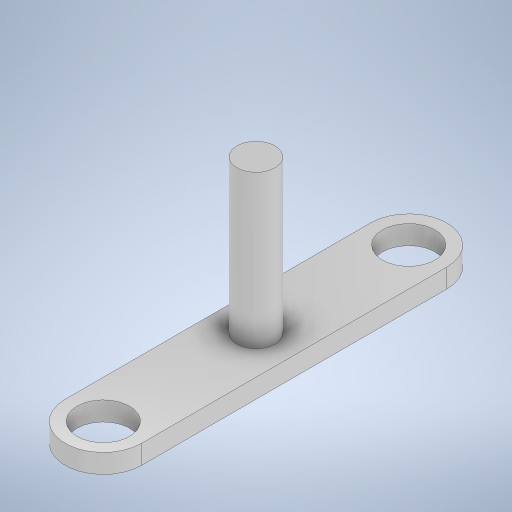
# Autodesk Inventor part: Torqueing_Bar
Saved by Autodesk Inventor 2024 (Build 280153000, 153)
## iProperties
Created: 2023-10-06
Part Number: Torqueing_Bar
Material: Generic
Document SubType Name: Modeling
Designer: tangl
Density: 1 g/cm^3
Appearance: Aluminum - Polished
Author: tangl
Autodesk Inventor part; units mm, degrees
ref_plane "YZ Plane" through (0, 0, 0) normal (1, 0, 0) x (0, 1, 0)
ref_plane "XZ Plane" through (0, 0, 0) normal (0, 1, 0) x (-1, 0, 0)
ref_plane "XY Plane" through (0, 0, 0) normal (0, 0, 1) x (1, 0, 0)
sketch "Sketch10" plane through (0, 0, 0) normal (0, 1, 0) x (-1, 0, 0)
  circle A0 centre (0, 0) radius 8.7376
  arc A1 (-12.7, 0) -> (12.7, 0) centre (0, 0) ccw
  line L0 (0, 0) -> (0, 101.6) construction
  circle A2 centre (0, 101.6) radius 8.7376
  arc A3 (12.7, 101.6) -> (-12.7, 101.6) centre (0, 101.6) ccw
  line L1 (12.7, 101.6) -> (12.7, 0)
  line L2 (-12.7, 0) -> (-12.7, 101.6)
  dimension "d70" = 17.4752
  dimension "d71" = 25.4
  dimension "d72" = 101.6
  dimension "d74" = 17.4752
  dimension "d75" = 25.4
  dimension "d76" = 101.6
  dimension "d78" = 12.7
  constraints: 6 end point, 4 centre point, 4 coincident, 4 point on circle, 2 vertical, 1 tangent
  measures "d70" diameter of A0
  measures "d71" diameter of A1
  measures "d72" distance of L0.start L0.end
  measures "d74" diameter of A2
  measures "d75" diameter of A3
  measures "d76" distance of L2.end L2.start
  measures "d78" distance from line of L1 point (0, 0)
extrude "Extrusion13" add sketch "Sketch10" along normal blind 6.35
sketch "Sketch11" plane through (0, 6.35, 0) normal (0, 1, 0) x (1, 0, 0)
  circle A0 centre (0, -50.8) radius 6.35
  line L0 (-12.7, 0) -> (-12.7, -101.6) projected
  point P0 (0, 0)
  dimension "d81" = 12.7
  dimension "d82" = 50.8
  dimension "d83" = 12.7
  constraints: 1 centre point
  measures "d81" diameter of A0
  measures "d82" distance of point (0, 0) A0.centre
  measures "d83" distance from line of L0 A0.centre
extrude "Extrusion14" add sketch "Sketch11" along normal blind 50.8
body "Solid7"
